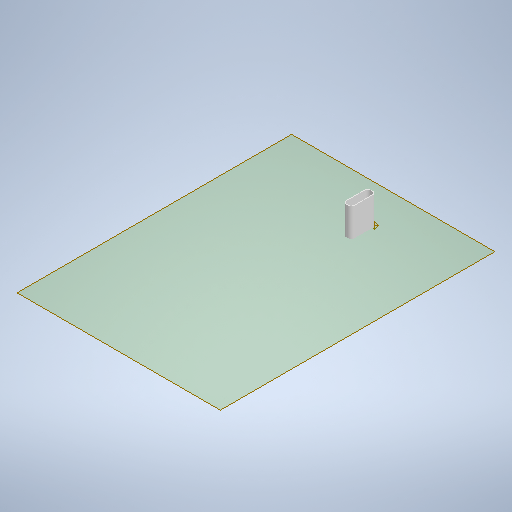
# Autodesk Inventor part: Camera_Assembly_Electrical
Saved by Autodesk Inventor 2025.1 (Build 291241000, 241)
## iProperties
Created: 2024-11-07
Part Number: Camera_Assembly_Electrical
Material: Generisch
Document SubType Name: Modeling
Designer: Kai Altwicker
Categories: <MemberInstance><Categories><Category DisplayName="" Mnemonic="CABLEANDHARNESS" InternalName="e4a7e005-5e42-4d16-b293-125e7f0d0512"><Category DisplayName="" Mnemonic="CONNECTORS" InternalName="6f634eba-a678-4820-a31d-2c2d5ee6728e"><CategoryParameter DisplayName="" Mnemonic="REFDES" InternalName="c3740e8c-60ab-4d5d-8584-52b73222f2f0"/><Category DisplayName="" Mnemonic="DISCRETEWIRE" InternalName="9a3407de-09b2-4cdb-8c40-9708d5144a28"/></Category></Category></Categories><FamilyTemplate><FamilyTemplateParameters></FamilyTemplateParameters></FamilyTemplate><CategoryParameterMap><ParamToTemplateMap><ParamToTemplate CategoryParameter="//CategoryParameter[@InternalName='c3740e8c-60ab-4d5d-8584-52b73222f2f0']" ConstantValue=""/></ParamToTemplateMap></CategoryParameterMap></MemberInstance>
Density: 1 g/cm^3
Appearance: Vorgabe
Author: Kai Altwicker
Autodesk Inventor part; units mm, degrees
ref_plane "YZ Plane" through (0, 0, 0) normal (1, 0, 0) x (0, 1, 0)
ref_plane "XZ Plane" through (0, 0, 0) normal (0, 1, 0) x (-1, 0, 0)
ref_plane "XY Plane" through (0, 0, 0) normal (0, 0, 1) x (1, 0, 0)
ref_plane "Arbeitsebene1" through (-28.1717, -118.9029, 44.8795) normal (0, -1, 0) x (1, 0, 0)
sketch "Skizze1" plane through (-28.1717, -118.9029, 44.8795) normal (0, -1, 0) x (1, 0, 0)
  line L0 (-16.24, -39.62) -> (-16.8, -39.62) projected
  arc A0 (-16.24, -39.62) -> (-14.94, -38.32) centre (-16.24, -38.32) ccw projected
  line L1 (-14.94, -38.32) -> (-14.94, -31.98) projected
  arc A1 (-14.94, -31.98) -> (-16.24, -30.68) centre (-16.24, -31.98) ccw projected
  line L2 (-16.24, -30.68) -> (-16.8, -30.68) projected
  arc A2 (-16.8, -30.68) -> (-18.1, -31.98) centre (-16.8, -31.98) ccw projected
  line L3 (-18.1, -38.32) -> (-18.1, -31.98) projected
  arc A3 (-18.1, -38.32) -> (-16.8, -39.62) centre (-16.8, -38.32) ccw projected
  arc A4 (-16.8, -30.98) -> (-17.8, -31.98) centre (-16.8, -31.98) ccw projected
  line L4 (-16.24, -30.98) -> (-16.8, -30.98) projected
  arc A5 (-15.24, -31.98) -> (-16.24, -30.98) centre (-16.24, -31.98) ccw projected
  line L5 (-15.24, -31.98) -> (-15.24, -38.32) projected
  arc A6 (-16.24, -39.32) -> (-15.24, -38.32) centre (-16.24, -38.32) ccw projected
  line L6 (-16.8, -39.32) -> (-16.24, -39.32) projected
  arc A7 (-17.8, -38.32) -> (-16.8, -39.32) centre (-16.8, -38.32) ccw projected
  line L7 (-17.8, -38.32) -> (-17.8, -31.98) projected
  point P0 (28.1717, -44.8795)
extrude "Extrusion1" add sketch "Skizze1" against normal blind 10
equation "\"d_tol\" = 0.3"
equation "\"d_wand\" = 1.5"
equation "\"r_rasp_pi\" = 3"
equation "\"D_oct\" = 3621.32034"
equation "\"d_traeger\" = 625"
equation "\"l_rasp_pi\" = 85"
equation "\"w_kamera_vert\" = 41deg"
equation "\"w_kamera_hori\" = 66deg"
equation "\"D_hexadeca\" = 7541.00924"
equation "\"b_rasp_pi\" = 56"
